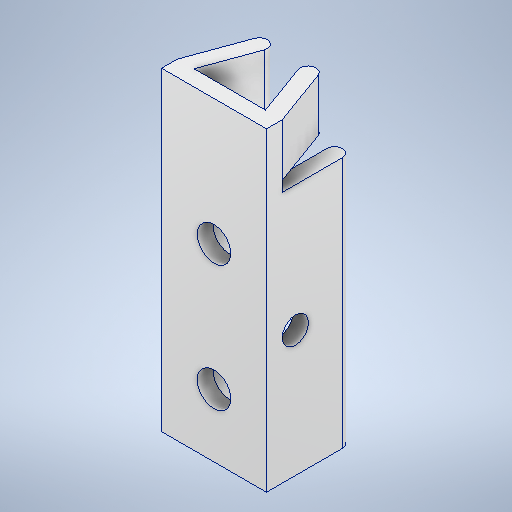
# Autodesk Inventor part: y_holder
Saved by Autodesk Inventor 2025 (Build 290162000, 162)
## iProperties
Created: 2024-04-25
Part Number: y_holder
Material: Hliník 6061
Document SubType Name: Modeling
Designer: rader
Density: 2.7 g/cm^3
Appearance: Hliník – plochý
Author: rader
Autodesk Inventor part; units mm, degrees
ref_plane "YZ Plane" through (0, 0, 0) normal (1, 0, 0) x (0, 1, 0)
ref_plane "XZ Plane" through (0, 0, 0) normal (0, 1, 0) x (-1, 0, 0)
ref_plane "XY Plane" through (0, 0, 0) normal (0, 0, 1) x (1, 0, 0)
sketch "Náčrt1" plane through (0, 0, 0) normal (0, 0, 1) x (1, 0, 0)
  line L0 (-5, 8) -> (-5, 0)
  line L1 (-5, 0) -> (5, 0)
  line L2 (5, 0) -> (5, 8)
  line L3 (5, 8) -> (3.5, 8)
  line L4 (3.5, 8) -> (3.5, 1.5)
  line L5 (3.5, 1.5) -> (-3.5, 1.5)
  line L6 (-3.5, 1.5) -> (-3.5, 8)
  line L7 (-3.5, 8) -> (-5, 8)
  line L8 (-7, 0) -> (7, 0) projected
  line L9 (0, 9.6) -> (0, -1.6) projected
  point P0 (0, 0)
  dimension "d0" = 10
  dimension "d1" = 8
  dimension "d2" = 1.5
  dimension "d3" = 1.5
  dimension "d4" = 1.5
  constraints: 16 end point, 7 perpendicular, 1 collinear, 1 point on line, 1 vertical, 1 other
  measures "d0" distance of L0.end L1.end
  measures "d1" distance of L0.start L0.end
  measures "d2" distance between parallel lines of L1 L5
  measures "d3" distance between parallel lines of L4 L2
  measures "d4" distance between parallel lines of L0 L6
extrude "Vysunutí1" add sketch "Náčrt1" along normal mid plane 24
sketch "Náčrt2" plane through (0, 0, 12) normal (0, 0, 1) x (1, 0, 0)
  line L0 (-5, 8) -> (-5, 0) projected
  line L1 (-5, 0) -> (5, 0) projected
  line L2 (5, 0) -> (5, 8) projected
  line L3 (5, 8) -> (3.5, 8) projected
  line L4 (3.5, 8) -> (3.5, 1.5) projected
  line L5 (3.5, 1.5) -> (-3.5, 1.5) projected
  line L6 (-3.5, 1.5) -> (-3.5, 8) projected
  line L7 (-3.5, 8) -> (-5, 8) projected
  line L8 (-5, 0) -> (5, 0)
  line L9 (5, 0) -> (5, 1.5)
  line L10 (5, 1.5) -> (-5, 1.5)
  line L11 (-5, 1.5) -> (-5, 0)
  line L12 (3.5, 1.5) -> (-3.5, 1.5) projected
  point P0 (0, 0)
  constraints: 8 end point, 2 parallel, 1 collinear, 1 horizontal, 1 perpendicular, 1 point on line
extrude "Vysunutí2" add sketch "Náčrt2" along normal blind 1 contours L10 L5 L2 L1 L0
sketch "Náčrt3" plane through (0, 0, 13) normal (0, 0, 1) x (1, 0, 0)
  line L0 (-5, 1.5) -> (-5, 0) projected
  line L1 (-5, 0) -> (5, 0) projected
  line L2 (5, 0) -> (5, 1.5) projected
  line L3 (5, 1.5) -> (-5, 1.5) projected
  line L4 (-5, 1.5) -> (-5, 0)
  line L5 (5, 0) -> (-5, 0)
  line L6 (3.5, 1.5) -> (5, 1.5) projected
  line L7 (5, 1.5) -> (5, 0)
  line L8 (-5, 1.5) -> (-2.7769, 7.608)
  line L9 (-5, 1.5) -> (1.5, 1.5) construction
  line L10 (-2.7769, 7.608) -> (-1.3673, 7.095)
  line L11 (-1.3673, 7.095) -> (-3.4037, 1.5)
  line L12 (0, 9.6) -> (0, -1.6) projected
  line L13 (5, 1.5) -> (2.7769, 7.608)
  line L14 (2.7769, 7.608) -> (1.3673, 7.095)
  line L15 (1.3673, 7.095) -> (3.4037, 1.5)
  line L16 (-3.4037, 1.5) -> (3.4037, 1.5)
  line L17 (-3.4037, 1.5) -> (3.4037, 1.5)
  point P0 (0, 0)
  dimension "d9" = 6.5
  dimension "d10" = 70
  dimension "d11" = 1.5
  constraints: 24 end point, 4 collinear, 3 symmetric about line, 2 perpendicular, 1 equal length, 1 horizontal, 1 point on line
  measures "d9" distance of L0.start L8.end
  measures "d10" angle of L9 L8
  measures "d11" distance of L8.end L10.end
extrude "Vysunutí3" add sketch "Náčrt3" along normal blind 5
fillet "Zaoblení1" radius 0.75 8 edges at (-3.5, 8, 0) (-5, 8, 0) (-2.7769, 7.608, 15.5) (-1.3673, 7.095, 15.5) (1.3673, 7.095, 15.5) (2.7769, 7.608, 15.5) (3.5, 8, 0) (5, 8, 0)
sketch "Náčrt4" plane through (5, 0, 18) normal (1, 0, 0) x (0, 0, -1)
  line L0 (6, 7.25) -> (30, 7.25) projected
  line L1 (6, 1.5) -> (6, 7.25) projected
  line L2 (6, 1.5) -> (5, 1.5) projected
  line L3 (5, 1.5) -> (0, 1.5) projected
  line L4 (0, 0) -> (0, 1.5) projected
  line L5 (30, 0) -> (0, 0) projected
  line L6 (30, 7.25) -> (30, 0) projected
  point P0 (18, 0)
  point P1 (18, 2.75)
  dimension "d15" = 12
  dimension "d16" = 2.75
  measures "d15" distance from line of L6 point (18, 2.75)
  measures "d16" distance from line of L5 point (18, 2.75)
hole "Díra1" at (5, 2.75, 0) direction (-1, 0, 0) diameter 2.5 end through all
sketch "Náčrt5" plane through (-3.5, 1.5, -12) normal (0, 1, 0) x (1, 0, 0)
  line L0 (7, 0) -> (7, -12) projected
  line L1 (0, 0) -> (7, 0) projected
  line L2 (0, 0) -> (0, -12) projected
  line L3 (0, -12) -> (0, -24) projected
  line L4 (-1.5, -24) -> (0, -24) projected
  line L5 (-1.5, -24) -> (-1.5, -25) projected
  line L6 (0.0963, -25) -> (-1.5, -25) projected
  line L7 (0.0963, -25) -> (0.0963, -30) projected
  line L8 (6.9037, -30) -> (0.0963, -30) projected
  line L9 (6.9037, -25) -> (6.9037, -30) projected
  line L10 (8.5, -25) -> (6.9037, -25) projected
  line L11 (8.5, -24) -> (8.5, -25) projected
  line L12 (7, -24) -> (8.5, -24) projected
  line L13 (7, -12) -> (7, -24) projected
  line L14 (-1.5, 0) -> (-1.5, -24) projected
  point P0 (3.5, -12)
  point P1 (3.5, -6)
  point P2 (3.5, -18)
  dimension "d24" = 5
  dimension "d25" = 6
  dimension "d26" = 12
  measures "d24" distance from line of L14 point (3.5, -6)
  measures "d25" distance from line of L1 point (3.5, -6)
  measures "d26" distance of point (3.5, -18) point (3.5, -6)
hole "Díra2" at (0, 1.5, -6) at (0, 1.5, 6) direction (0, -1, 0) diameter 3.2 end through all
